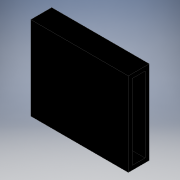
# Autodesk Inventor part: Bumper Support
Saved by Autodesk Inventor 2019.4 (Build 234330000, 330)
## iProperties
Created: 2019-12-12
Part Number: Bumper Support
Material: Aluminum 6061
Document SubType Name: Modeling
Designer: admin
Density: 2.7 g/cm^3
Appearance: Anodized - Black
Author: admin
Autodesk Inventor part; units mm, degrees
ref_plane "YZ Plane" through (0, 0, 0) normal (1, 0, 0) x (0, 1, 0)
ref_plane "XZ Plane" through (0, 0, 0) normal (0, 1, 0) x (-1, 0, 0)
ref_plane "XY Plane" through (0, 0, 0) normal (0, 0, 1) x (1, 0, 0)
sketch "Sketch1" plane through (0, 0, 0) normal (1, 0, 0) x (0, 1, 0)
  line L0 (-30, 7.5) -> (30, 7.5)
  line L1 (30, 7.5) -> (30, -7.5)
  line L2 (30, -7.5) -> (-30, -7.5)
  line L3 (-30, -7.5) -> (-30, 7.5)
  line L4 (-30, 7.5) -> (30, -7.5) construction
  line L5 (30, 7.5) -> (-30, -7.5) construction
  line L6 (27, -4.5) -> (27, 4.5)
  line L7 (27, 4.5) -> (-27, 4.5)
  line L8 (-27, 4.5) -> (-27, -4.5)
  line L9 (-27, -4.5) -> (27, -4.5)
  point P0 (0, 0)
  dimension "d0" = 60
  dimension "d1" = 15
  dimension "d2" = 3
  constraints: 20 end point, 4 parallel, 2 midpoint, 2 perpendicular, 1 horizontal, 3 other
  measures "d0" distance of L1.end L2.end
  measures "d1" distance of L0.end L1.end
  measures "d2" distance between parallel lines of L1 L6
extrude "Extrusion1" add sketch "Sketch1" along normal blind 70
body "Solid1"
